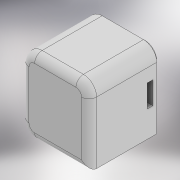
# Autodesk Inventor part: Cap
Saved by Autodesk Inventor 2020 (Build 240168000, 168)
## iProperties
Created: 2022-04-06
Part Number: Cap
Material: 일반
Document SubType Name: Modeling
Designer: Knowblesse
Density: 1 g/cm^3
Appearance: 기본값
Author: Knowblesse
## iProperties of the stored document _3D 인쇄.ipt
Created: 2022-04-06
Part Number: _3D 인쇄
Material: 일반
Document SubType Name: Modeling
Designer: Knowblesse
Density: 1 g/cm^3
Appearance: 기본값
Author: Knowblesse
Autodesk Inventor part; units mm, degrees
ref_plane "YZ Plane" through (0, 0, 0) normal (1, 0, 0) x (0, 1, 0)
ref_plane "XZ Plane" through (0, 0, 0) normal (0, 1, 0) x (-1, 0, 0)
ref_plane "XY Plane" through (0, 0, 0) normal (0, 0, 1) x (1, 0, 0)
sketch "스케치1" plane through (0, 0, 0) normal (0, 0, 1) x (1, 0, 0)
  line L0 (-5.5, -8.5) -> (7.5, -8.5)
  line L1 (7.5, -8.5) -> (7.5, 6.5)
  line L2 (5.5, 8.5) -> (-5.5, 8.5)
  line L3 (-7.5, 6.5) -> (-7.5, -6.5)
  line L4 (-7.5, -8.5) -> (7.5, 8.5) construction
  line L5 (7.5, -8.5) -> (-7.5, 8.5) construction
  arc A0 (-5.5, 8.5) -> (-7.5, 6.5) centre (-5.5, 6.5) ccw
  arc A1 (7.5, 6.5) -> (5.5, 8.5) centre (5.5, 6.5) ccw
  arc A2 (-7.5, -6.5) -> (-5.5, -8.5) centre (-5.5, -6.5) ccw
  line L6 (-5.5, 10) -> (5.5, 10)
  arc A3 (9, 6.5) -> (5.5, 10) centre (5.5, 6.5) ccw
  line L7 (9, 6.5) -> (9, -10)
  line L8 (9, -10) -> (-5.5, -10)
  arc A4 (-9, -6.5) -> (-5.5, -10) centre (-5.5, -6.5) ccw
  line L9 (-9, -6.5) -> (-9, 6.5)
  arc A5 (-5.5, 10) -> (-9, 6.5) centre (-5.5, 6.5) ccw
  point P0 (0, 0)
  dimension "d0" = 17
  dimension "d1" = 15
  dimension "d2" = 2
  dimension "d3" = 1.5
  constraints: 20 end point, 12 point on circle, 6 centre point, 6 point on line, 6 tangent, 4 parallel, 2 equal radius, 2 midpoint, 2 perpendicular, 1 horizontal, 6 other
  measures "d0" distance of L0.end L4.end
  measures "d1" distance of L4.end L5.end
  measures "d2" radius of A0
  measures "d3" distance between parallel lines of L2 L6
extrude "돌출1" add sketch "스케치1" along normal blind 17
sketch "스케치2" plane through (0, 0, 17) normal (0, 0, 1) x (1, 0, 0)
  line L0 (-5.5, -10) -> (9, -10) projected
  line L1 (9, -10) -> (9, 6.5) projected
  arc A0 (9, 6.5) -> (5.5, 10) centre (5.5, 6.5) ccw projected
  line L2 (5.5, 10) -> (-5.5, 10) projected
  arc A1 (-5.5, 10) -> (-9, 6.5) centre (-5.5, 6.5) ccw projected
  line L3 (-9, 6.5) -> (-9, -6.5) projected
  arc A2 (-9, -6.5) -> (-5.5, -10) centre (-5.5, -6.5) ccw projected
  point P0 (0, 0)
extrude "돌출2" add sketch "스케치2" along normal blind 1.5
sketch "스케치3" plane through (-9, -6.5, 0) normal (-1, 0, 0) x (0, 0, 1)
  line L0 (0, 13) -> (0, 0) projected
  line L1 (3, 3.5) -> (1.5, 3.5)
  line L2 (1.5, 3.5) -> (1.5, 9.5)
  line L3 (1.5, 9.5) -> (3, 9.5)
  line L4 (3, 9.5) -> (3, 3.5)
  point P0 (0, 6.5)
  point P1 (0, 6.5)
  point P2 (1.5, 6.5)
  dimension "d8" = 6
  dimension "d9" = 1.5
  dimension "d10" = 1.5
  constraints: 8 end point, 2 midpoint, 2 parallel, 1 horizontal, 1 horizontal alignment, 1 perpendicular
  measures "d8" distance of L1.end L2.end
  measures "d9" distance of L2.end L3.end
  measures "d10" distance between parallel lines of L2 L0
extrude "돌출3" cut sketch "스케치3" against normal through all
fillet "모깎기1" radius 2 7 edges at (-7.9749, -8.9749, 18.5) (1.75, -10, 18.5) (-7.9749, 8.9749, 18.5) (0, 10, 18.5) (7.9749, 8.9749, 18.5) (9, -1.75, 18.5) (-9, 0, 18.5)
chamfer "모따기1" distance 0.5 angle 45 7 edges at (1.75, -10, 0) (-7.9749, -8.9749, 0) (-9, 0, 0) (-7.9749, 8.9749, 0) (0, 10, 0) (7.9749, 8.9749, 0) (9, -1.75, 0)
